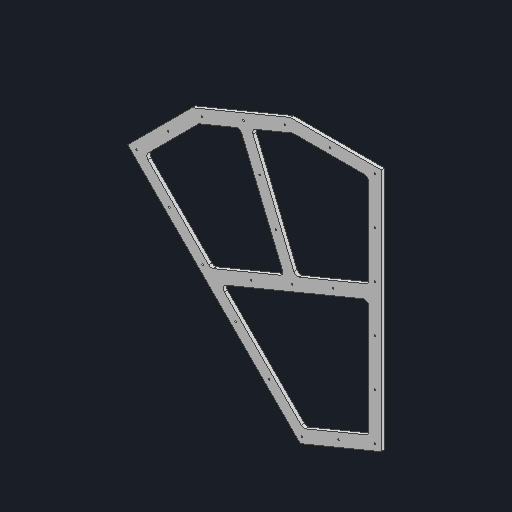
# Autodesk Inventor part: DMF 01 56 Крепление сетки к кассете v2.1
Saved by Autodesk Inventor 2026.2 (Build 302298000, 298)
## iProperties
Created: 2024-05-05
Part Number: DMF 01 56 Крепление сетки к кассете v2.1
Material: Generic
Document SubType Name: Modeling
Designer: pokla
Density: 1 g/cm^3
Appearance: Default
Author: pokla
Autodesk Inventor part; units mm, degrees
ref_plane "YZ Plane" through (0, 0, 0) normal (1, 0, 0) x (0, 1, 0)
ref_plane "XZ Plane" through (0, 0, 0) normal (0, 1, 0) x (-1, 0, 0)
ref_plane "XY Plane" through (0, 0, 0) normal (0, 0, 1) x (1, 0, 0)
sketch "Sketch1" plane through (0, 0, 0) normal (0, 0, 1) x (1, 0, 0)
  line L0 (0, 278.716) -> (197.082, 197.082) construction
  line L1 (197.082, 197.082) -> (278.716, 0) construction
  line L2 (278.716, 0) -> (197.082, -197.082) construction
  line L3 (197.082, -197.082) -> (0, -278.716) construction
  line L4 (0, -278.716) -> (-197.082, -197.082) construction
  line L5 (-197.082, -197.082) -> (-278.716, 0) construction
  line L6 (-278.716, 0) -> (-197.082, 197.082) construction
  line L7 (-197.082, 197.082) -> (0, 278.716)
  line L8 (-197.082, 197.082) -> (0, 278.716)
  line L9 (-461.6493, 774.8136) -> (-221.4406, 874.3113)
  line L10 (-98.541, 237.899) -> (-341.545, 824.5625) construction
  line L11 (-221.4406, 874.3113) -> (0, 874.3113)
  line L12 (0, 874.3113) -> (0, 278.716)
  line L13 (-461.6493, 774.8136) -> (-618.2315, 618.2315)
  line L14 (-618.2315, 618.2315) -> (-197.082, 197.082)
  point P0 (0, 0)
  point P1 (0, 0)
  dimension "d0" = 515
  dimension "d2" = 260
  dimension "d3" = 635
  constraints: 30 end point, 2 midpoint, 1 coincident, 1 horizontal, 1 parallel, 1 perpendicular, 1 symmetric about line, 1 vertical, 1 vertical alignment, 17 other
  measures "d0" distance between parallel lines of L5 L1
  measures "d2" distance of L9.start L9.end
  measures "d3" distance of L10.end L10.start
extrude "Extrusion1" add sketch "Sketch1" along normal mid plane 8
sketch "Sketch2" plane through (0, 0, 4) normal (0, 0, 1) x (1, 0, 0)
  line L0 (-221.4406, 874.3113) -> (-461.6493, 774.8136) projected
  line L1 (-461.6493, 774.8136) -> (-618.2315, 618.2315) projected
  line L2 (-236.7713, 532.4196) -> (-415.8262, 458.2526)
  line L3 (-197.082, 197.082) -> (0, 278.716) projected
  line L4 (-98.541, 237.899) -> (-341.545, 824.5625) construction
  line L5 (-618.2315, 618.2315) -> (-197.082, 197.082) projected
  line L6 (-415.8262, 458.2526) -> (-575.8051, 618.2315)
  line L7 (-575.8051, 618.2315) -> (-444.6557, 749.3809)
  line L8 (-444.6557, 749.3809) -> (-343.9227, 791.1058)
  line L9 (-236.7713, 532.4196) -> (-343.9227, 791.1058)
  line L10 (-209.0549, 543.9001) -> (-30, 618.067)
  line L11 (-30, 618.067) -> (-30, 844.3113)
  line L12 (-30, 844.3113) -> (-215.4733, 844.3113)
  line L13 (-215.4733, 844.3113) -> (-316.2063, 802.5863)
  line L14 (-209.0549, 543.9001) -> (-316.2063, 802.5863)
  line L15 (0, 278.716) -> (0, 874.3113) projected
  line L16 (-415.8262, 458.2526) -> (-30, 618.067) construction
  line L17 (-392.8652, 435.2916) -> (-30, 585.5953)
  line L18 (-190.043, 232.4694) -> (-30, 298.7614)
  line L19 (-30, 298.7614) -> (-30, 585.5953)
  line L20 (-190.043, 232.4694) -> (-392.8652, 435.2916)
  point P0 (0, 0)
  dimension "d11" = 30
  dimension "d12" = 280
  dimension "d13" = 30
  dimension "d14" = 30
  dimension "d15" = 15
  dimension "d21" = 30
  dimension "d22" = 30
  dimension "d23" = 30
  dimension "d24" = 30
  constraints: 32 end point, 5 parallel, 5 symmetric about line, 2 midpoint, 1 collinear
  measures "d11" distance between parallel lines of L5 L6
  measures "d12" distance between parallel lines of L8 L2
  measures "d13" distance between parallel lines of L0 L8
  measures "d14" distance between parallel lines of L1 L7
  measures "d15" distance between parallel lines of L9 L4
  measures "d21" distance between parallel lines of L16 L17
  measures "d22" distance between parallel lines of L5 L20
  measures "d23" distance between parallel lines of L19 L15
  measures "d24" distance between parallel lines of L18 L3
extrude "Extrusion2" cut sketch "Sketch2" against normal up to surface (8 mm away)
fillet "Fillet1" radius 10 12 edges at (-575.8051, 618.2315, 0) (-343.9227, 791.1058, 0) (-236.7713, 532.4196, 0) (-415.8262, 458.2526, 0) (-316.2063, 802.5863, 0) (-30, 844.3113, 0) (-30, 618.067, 0) (-209.0549, 543.9001, 0) (-392.8652, 435.2916, 0) (-30, 585.5953, 0) (-30, 298.7614, 0) (-190.043, 232.4694, 0)
sketch "Sketch5" plane through (0, 0, 4) normal (0, 0, 1) x (1, 0, 0)
  line L0 (-221.4406, 874.3113) -> (-461.6493, 774.8136) projected
  line L1 (0, 874.3113) -> (-221.4406, 874.3113) projected
  line L2 (-461.6493, 774.8136) -> (-618.2315, 618.2315) projected
  line L3 (-618.2315, 618.2315) -> (-197.082, 197.082) projected
  line L4 (-197.082, 197.082) -> (0, 278.716) projected
  line L5 (0, 278.716) -> (0, 874.3113) projected
  line L6 (-15, 859.3113) -> (-218.4569, 859.3113) construction
  line L7 (-218.4569, 859.3113) -> (-453.1525, 762.0973) construction
  line L8 (-453.1525, 762.0973) -> (-597.0183, 618.2315) construction
  line L9 (-597.0183, 618.2315) -> (-193.5625, 214.7757) construction
  line L10 (-193.5625, 214.7757) -> (-15, 288.7387) construction
  line L11 (-15, 288.7387) -> (-15, 859.3113) construction
  line L12 (-379.0384, 441.0189) -> (-43.8268, 579.868) projected
  line L13 (-212.8817, 553.1389) -> (-312.3794, 793.3476) projected
  line L14 (-419.3457, 440.5589) -> (-15, 608.0444) construction
  line L15 (-217.1728, 524.3016) -> (-335.8047, 810.7043) construction
  circle A0 centre (-335.8047, 810.7043) radius 2
  circle A1 centre (-217.1728, 524.3016) radius 2
  circle A2 centre (-296.262, 715.2398) radius 2
  circle A3 centre (-256.7194, 619.7753) radius 2
  circle A4 centre (-597.0183, 618.2315) radius 2
  circle A5 centre (-516.2262, 537.4394) radius 2
  circle A6 centre (-435.4342, 456.6474) radius 2
  circle A7 centre (-354.6421, 375.8553) radius 2
  circle A8 centre (-273.8501, 295.0633) radius 2
  circle A9 centre (-193.0581, 214.2713) radius 2
  circle A10 centre (-317.4138, 482.7805) radius 2
  circle A11 centre (-104.2812, 251.7572) radius 2
  circle A12 centre (-519.2365, 696.0132) radius 2
  circle A13 centre (-437.4315, 768.6091) radius 2
  circle A14 centre (-15, 859.3113) radius 2
  circle A15 centre (-15, 745.0541) radius 2
  circle A16 centre (-15, 630.7969) radius 2
  circle A17 centre (-15, 516.5397) radius 2
  circle A18 centre (-15, 402.2825) radius 2
  circle A19 centre (-15, 288.0253) radius 2
  circle A20 centre (-116.9319, 565.8228) radius 2
  circle A21 centre (-125, 859.3113) radius 2
  circle A22 centre (-234.178, 852.7995) radius 2
  point P0 (0, 0)
  dimension "d32" = 15
  dimension "d33" = 15
  dimension "d34" = 15
  dimension "d35" = 4
  dimension "d37" = 103.33
  dimension "d38" = 103.33
  dimension "d43" = 114.2572
  dimension "d49" = 108.5
  dimension "d50" = 110
  dimension "d51" = 110
  constraints: 23 centre point, 16 end point, 9 symmetric about line, 8 equal radius, 7 point on line, 3 coincident, 3 midpoint, 2 parallel, 25 other
  measures "d32" distance between parallel lines of L5 L11
  measures "d33" distance between parallel lines of L12 L14
  measures "d34" distance between parallel lines of L13 L15
  measures "d35" diameter of A0
  measures "d37" distance of A2.centre A0.centre
  measures "d38" distance of A3.centre A2.centre
  measures "d43" distance of A4.centre A5.centre
  measures "d49" distance of A1.centre A10.centre
  measures "d50" distance of A12.centre A4.centre
  measures "d51" distance of A13.centre A0.centre
extrude "Extrusion4" cut sketch "Sketch5" against normal up to surface (8 mm away) contours A0 | A1 | A2 | A3 | A4 | A5 | A6 | A7 | A8 | A9 | A10 | A11 | A12 | A13 | A14 | A15 | A16 | A17 | A18 | A19 | A20 | A21 | A22
equation "\"d0\" = Барабан_размер_по_плоскостям"
equation "\"d2\" = Кассета_длина_грани"
equation "\"d3\" = Кассета_высота"
equation "\"d11\" = d13"
equation "\"d14\" = d13"
equation "\"d15\" = 0.5 * d13"
equation "\"d21\" = d13"
equation "\"d22\" = d13"
equation "\"d23\" = d13"
equation "\"d24\" = d13"
equation "\"Барабан_размер_по_плоскостям\" = 515"
equation "\"Кассета_длина_грани\" = 260"
equation "\"Кассета_высота\" = 635"
body "Solid1"
